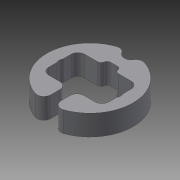
# Autodesk Inventor part: Aft Endcap Middle
Saved by Autodesk Inventor 2015 (Build 190159000, 159)
## iProperties
Created: 2015-04-23
Part Number: Aft Endcap Middle
Material: Generic
Document SubType Name: Modeling
Designer: JR
Density: 1 g/cm^3
Appearance: Default
Author: JR
Autodesk Inventor part; units mm, degrees
ref_plane "YZ Plane" through (0, 0, 0) normal (1, 0, 0) x (0, 1, 0)
ref_plane "XZ Plane" through (0, 0, 0) normal (0, 1, 0) x (-1, 0, 0)
ref_plane "XY Plane" through (0, 0, 0) normal (0, 0, 1) x (1, 0, 0)
sketch "Sketch1" plane through (0, 0, 0) normal (0, 0, 1) x (1, 0, 0)
  arc A0 (-1.7105, 10.9635) -> (1.7105, 10.9635) centre (0, 12) ccw
  arc A1 (-1.7105, 10.9635) -> (-4.0726, 11.818) centre (-3.421, 9.9271) ccw
  arc A2 (4.0726, 11.818) -> (1.7105, 10.9635) centre (3.421, 9.9271) ccw
  arc A3 (-6.75, 5.25) -> (-8.75, 3.25) centre (-6.75, 3.25) ccw
  arc A4 (8.75, 3.25) -> (6.75, 5.25) centre (6.75, 3.25) ccw
  arc A5 (-8.75, -3.25) -> (-6.75, -5.25) centre (-6.75, -3.25) ccw
  arc A6 (6.75, -5.25) -> (8.75, -3.25) centre (6.75, -3.25) ccw
  arc A7 (-8.85, 0.6538) -> (-8.85, -0.6538) centre (-7.5, 0) ccw
  arc A8 (8.85, -0.6538) -> (8.85, 0.6538) centre (7.5, 0) ccw
  line L0 (0, 6.25) -> (0, -6.25) construction
  line L1 (8.75, -3.25) -> (8.75, -1.0897)
  line L2 (8.75, 1.0897) -> (8.75, 3.25)
  line L3 (-8.75, 3.25) -> (-8.75, 1.0897)
  line L4 (-8.75, -1.0897) -> (-8.75, -3.25)
  line L5 (-1.5, -7.25) -> (-1.5, -9.8995)
  line L6 (1.5, -7.25) -> (1.5, -9.8995)
  line L7 (-7.5, 0) -> (7.5, 0) construction
  line L8 (-6.75, -5.25) -> (-3.5, -5.25)
  line L9 (3.5, -5.25) -> (6.75, -5.25)
  line L10 (-6.75, 5.25) -> (-6.75, -5.25) construction
  arc A9 (-1.5, -7.25) -> (-3.5, -5.25) centre (-3.5, -7.25) ccw
  arc A10 (3.5, -5.25) -> (1.5, -7.25) centre (3.5, -7.25) ccw
  arc A11 (-4.0726, 11.818) -> (-4.1667, -11.7851) centre (0, 0) ccw
  arc A12 (4.1667, -11.7851) -> (4.0726, 11.818) centre (0, 0) ccw
  arc A13 (-4.1667, -11.7851) -> (-1.5, -9.8995) centre (-3.5, -9.8995) ccw
  arc A14 (1.5, -9.8995) -> (4.1667, -11.7851) centre (3.5, -9.8995) ccw
  line L11 (-1, 7) -> (1, 7)
  line L12 (-2, 6) -> (-2, 6.25)
  line L13 (2, 6) -> (2, 6.25)
  line L14 (6.75, 5.25) -> (3, 5.25)
  line L15 (-3, 5.25) -> (-6.75, 5.25)
  arc A15 (-1, 7) -> (-2, 6) centre (-1, 6) ccw
  arc A16 (2, 6) -> (1, 7) centre (1, 6) ccw
  arc A17 (-3, 5.25) -> (-2, 6.25) centre (-3, 6.25) ccw
  arc A18 (2, 6.25) -> (3, 5.25) centre (3, 6.25) ccw
  arc A19 (-8.85, 0.6538) -> (-8.75, 1.0897) centre (-9.75, 1.0897) ccw
  arc A20 (-8.75, -1.0897) -> (-8.85, -0.6538) centre (-9.75, -1.0897) ccw
  arc A21 (8.75, 1.0897) -> (8.85, 0.6538) centre (9.75, 1.0897) ccw
  arc A22 (8.85, -0.6538) -> (8.75, -1.0897) centre (9.75, -1.0897) ccw
  line L16 (-8.75, 3.25) -> (8.75, 3.25) construction
  point P0 (0, 0)
  point P1 (-8.75, -0.8292)
  point P2 (-8.75, 0.8292)
  point P3 (8.75, 0.8292)
  point P4 (8.75, -0.8292)
  point P5 (-1.5, -12.4097)
  point P6 (1.5, -5.25)
  point P7 (1.5, -12.4097)
  point P8 (-1.5, -5.25)
  point P9 (-6.75, 0)
  point P10 (-2, 7)
  point P11 (2, 7)
  point P12 (0, 7)
  point P13 (0, 3.25)
  point P14 (0, 10)
  dimension "d3" = 4
  dimension "d5" = 2
  dimension "d6" = 2
  dimension "d7" = 3
  dimension "d8" = 3
  dimension "d10" = 15
  dimension "d11" = 3
  dimension "d15" = 2
  dimension "d16" = 2
  dimension "d17" = 2
  dimension "d18" = 7
  dimension "d19" = 4
  dimension "d20" = 10.5
  dimension "d21" = 1
  dimension "d22" = 1
  dimension "d25" = 12
  dimension "d26" = 12.5
  dimension "d27" = 17.5
  constraints: 53 point on circle, 43 tangent, 34 end point, 23 centre point, 15 point on line, 11 equal radius, 8 parallel, 8 perpendicular, 5 coincident, 5 horizontal, 5 midpoint, 4 vertical alignment, 3 horizontal alignment, 2 symmetric about line, 1 vertical
  measures "d3" diameter of A0
  measures "d5" radius of A1
  measures "d6" radius of A3
  measures "d7" diameter of A7
  measures "d8" diameter of A8
  measures "d10" distance of L7.end L7.start
  measures "d11" distance between parallel lines of L6 L5
  measures "d15" radius of A9
  measures "d16" radius of A10
  measures "d17" radius of A13
  measures "d18" distance from line of A11.centre L11
  measures "d19" distance of point (-2, 7) point (2, 7)
  measures "d20" distance between parallel lines of L9 L14
  measures "d21" radius of A15
  measures "d22" radius of A19
  measures "d25" distance of point (0, 0) A0.centre
  measures "d26" radius of A11
  measures "d27" distance of L3.start L2.end
extrude "Extrusion1" add sketch "Sketch1" along normal blind 6
body "Solid1"
